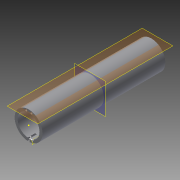
# Autodesk Inventor part: GripOuterTube
Saved by Autodesk Inventor 2014 SP1 (Build 180222100, 222)
## iProperties
Created: 2015-10-17
Part Number: GripOuterTube
Material: Generic
Document SubType Name: Modeling
Designer: anthony
Density: 1 g/cm^3
Appearance: Default
Author: anthony
Autodesk Inventor part; units mm, degrees
ref_plane "YZ Plane" through (0, 0, 0) normal (1, 0, 0) x (0, 1, 0)
ref_plane "XZ Plane" through (0, 0, 0) normal (0, 1, 0) x (-1, 0, 0)
sketch "Sketch1" plane through (0, 0, 0) normal (0, 1, 0) x (-1, 0, 0)
  circle A0 centre (0, 0) radius 11.75
  circle A1 centre (0, 0) radius 15
  line L0 (0, 0) -> (0, 22.6513) construction
  circle A2 centre (-2.7808, 13.0827) radius 1.3024
  line L1 (0, 0) -> (-2.7808, 13.0827) construction
  circle A3 centre (2.7808, 13.0827) radius 1.3024
  dimension "d0" = 23.5
  dimension "model_d6" = 30
  dimension "d9" = 13.375
  dimension "d10" = 168
  constraints: 4 centre point, 4 end point, 2 coincident, 1 symmetric about line, 1 vertical, 1 other
  measures "d0" diameter of A0
  measures "model_d6" diameter of A1
  measures "d9" distance of point (0, 0) L1.end
  measures "d10" angle of L0 L1
extrude "Extrusion1" add sketch "Sketch1" along normal blind 132
sketch "Sketch2" plane through (0, 0, 0) normal (0, -1, 0) x (1, 0, 0)
  circle A0 centre (0, 0) radius 11.75 projected
  circle A1 centre (0, 0) radius 15 projected
  line L0 (0, 0) -> (0, -41.0881) construction
  line L1 (0, 0) -> (-2.032, -24.3273) construction
  line L2 (-0.978, -11.7092) -> (-1.2486, -14.9479)
  line L3 (0, 0) -> (2.032, -24.3273) construction
  line L4 (0.978, -11.7092) -> (1.2486, -14.9479)
  arc A2 (-0.978, -11.7092) -> (0.978, -11.7092) centre (0, 0) ccw
  arc A3 (-1.2486, -14.9479) -> (1.2486, -14.9479) centre (0, 0) ccw
  dimension "d13" = 4.775
  constraints: 10 end point, 4 point on circle, 4 point on line, 3 symmetric about line, 2 centre point, 2 coincident, 1 vertical, 4 other
  measures "d13" angle of L1 L0
extrude "Extrusion2" cut sketch "Sketch2" against normal blind 8 contours A0 L4 A1 L2 picked at (0.1088, -13.9113)
sketch "Sketch3" plane through (0.978, 0, -11.7092) normal (-0.9965298, 0, -0.0832369) x (-0.0832369, 0, 0.9965298)
  circle A0 centre (-1.875, 2) radius 1
  point P0 (11.75, 0)
  dimension "d16" = 2
  constraints: 1 centre point
  measures "d16" diameter of A0
extrude "Extrusion3" cut sketch "Sketch3" against normal up to next
extrude "Extrusion4" cut sketch "Sketch3" along normal blind 4.25
thread "Thread1" size "M2x0.4" class "6H" standard "ANSI Metric M Profile" full length
ref_plane "Work Plane1" through (3.9676, 0, -11.4595) normal (-0.9965298, 0, -0.0832369) x (-0.0832369, 0, 0.9965298)
sketch "Sketch4" plane through (3.9676, 0, -11.4595) normal (-0.9965298, 0, -0.0832369) x (-0.0832369, 0, 0.9965298)
  circle A0 centre (-1.875, 2) radius 1 construction
  circle A1 centre (-1.875, 2) radius 1 projected
  circle A2 centre (-1.875, 2) radius 1.5
  point P0 (11.75, 0)
  dimension "d24" = 2
  dimension "d25" = 3
  constraints: 1 centre point, 1 coincident
  measures "d24" diameter of A0
  measures "d25" diameter of A2
extrude "Extrusion5" cut sketch "Sketch4" against normal up to next
ref_plane "Work Plane2" through (0, 66, 0) normal (0, 1, 0) x (1, 0, 0)
mirror "Mirror1" about plane through (0, 66, 0) normal (0, 1, 0) of "Extrusion5", "Extrusion2", "Extrusion4", "Extrusion3"
thread "Thread2" size "M2x0.4" class "6H" standard "ANSI Metric M Profile" full length
ref_plane "Work Plane4" through (0, 0, 13) normal (0, 0, 1) x (1, 0, 0)
sketch "Sketch6" plane through (0, 0, 13) normal (0, 0, 1) x (1, 0, 0)
  line L0 (-4.0832, 132) -> (-1.4785, 132) projected
  line L1 (-1.4785, 0) -> (-4.0832, 0) projected
  line L2 (-2.7808, 0) -> (-2.7808, 8.8616) construction
  circle A0 centre (-2.7808, 5.2335) radius 1.3031
  line L3 (4.0832, 0) -> (1.4785, 0) construction
  circle A1 centre (2.7288, 5.2335) radius 1.3024
  point P0 (0, 0)
  constraints: 2 centre point, 2 end point, 1 midpoint, 1 perpendicular, 1 point on line
extrude "Extrusion6" cut sketch "Sketch6" against normal up to next
ref_plane "Work Plane3" through (3.9676, 132, -11.4595) normal (0.9965298, 0, 0.0832369) x (-0.0832369, 0, 0.9965298)
equation "\"d0\" = d1"
equation "\"model_d6\" = d2"
equation "\"d9\" = rco0"
equation "\"d11\" = l1"
equation "\"d13\" = rebate_arc_angle"
equation "\"d14\" = rebate_depth"
equation "\"d17\" = rebate_depth"
equation "\"d1\" = 23.5"
equation "\"d2\" = 30"
equation "\"l1\" = 132"
equation "\"d3\" = 34"
equation "\"d4\" = 23.5"
equation "\"d5\" = 19"
equation "\"d6\" = 2.2"
equation "\"rco0\" = 13.375"
equation "\"rcod0\" = 12deg"
equation "\"rebate_arc_angle\" = 4.77465deg"
equation "\"rebate_arc\" = 5"
equation "\"rebate_depth\" = 8"
equation "\"min_wall_thickness\" = 1"
equation "\"cap_slot_rebate_angle\" = 8.42585deg"
equation "\"cap_slot_rebate_depth_radius\" = 14.375"
equation "\"cap_slot_rebate_depth\" = 4"
body "Solid1"
